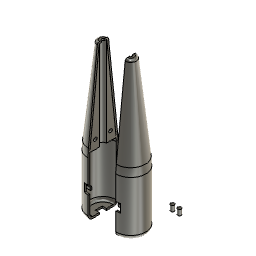
magic_wand_enclosure (Autodesk Fusion 360 design; units mm, degrees)
Autodesk Fusion 360 part; units mm, degrees
sketch "Sketch1" plane through (0, 0, 0) normal (0, 0, 1) x (1, 0, 0)
  circle A0 centre (0, 0) radius 19
  dimension "d1" = 38
  constraint coincident A0.centre origin
  measures "d1" diameter of A0
extrude "Extrude1" add sketch "Sketch1" along normal blind 82 makes body 1
sketch "Sketch2" plane through (0, 0, 82) normal (0, 0, 1) x (-1, 0, 0)
  circle A0 centre (0, 0) radius 19
  circle A1 centre (0, 0) radius 5
  dimension "d4" = 10
  constraint coincident A0.centre A1.centre
  measures "d4" diameter of A1
extrude "Extrude2" add sketch "Sketch2" along normal blind 128.5 contours A1 bodies 1
sketch "Sketch3" plane through (0, 0, 0) normal (0, 0, 1) x (1, 0, 0)
  circle A0 centre (70, 0) radius 19
  dimension "d7" = 38
  measures "d7" diameter of A0
extrude "Extrude3" add sketch "Sketch3" along normal blind 128.5 separate body makes body 2
sketch "Sketch4" plane through (0, 0, 128.5) normal (0, 0, 1) x (-1, 0, 0)
draft "Draft1" angle 6 neutral plane through (0, 0, 0) pull (0, 0, 1) 1 faces at (51.0944, 1.8918, 42.8333) on bodies 2
move_body "Move1" bodies 2 to x (1, 0, 0) y (0, 1, 0) z (0, 0, 1) at (-70, 0, 82)
combine "Combine1" operation add target body 2 tool bodies 1
fillet "Fillet1" radius 4 1 edges at (-17.7142, -6.8707, 0) on bodies 2
fillet "Fillet2" radius 0.8 1 edges at (-5.1223, -1.9868, 210.5) on bodies 2
fillet "Fillet3" radius 110 1 edges at (-17.7142, -6.8707, 82) on bodies 2
shell "Shell1" thickness 2.5 outward yes removed faces 0 bodies 2
sketch "Sketch5" plane through (0, 0, 0) normal (0, 0, 1) x (1, 0, 0)
  circle A0 centre (100, 0) radius 19
  dimension "d20" = 38
  measures "d20" diameter of A0
extrude "Extrude4" add sketch "Sketch5" along normal blind 128.5 separate body makes body 3
sketch "Sketch6" plane through (0, 0, 0) normal (0, 0, 1) x (1, 0, 0)
  circle A0 centre (150, 0) radius 5
  dimension "d23" = 10
  measures "d23" diameter of A0
extrude "Extrude5" add sketch "Sketch6" along normal blind 128.5 separate body makes body 4
move_body "Move2" bodies 4 to x (1, 0, 0) y (0, 1, 0) z (0, 0, 1) at (-50, 0, 0)
combine "Combine2" operation cut target body 3 tool bodies 4
draft "Draft2" angle 6 neutral plane through (0, 0, 0) pull (0, 0, 1) 1 faces at (81.0944, 1.8918, 42.8333) on bodies 3
move_body "Move3" bodies 3 to x (1, 0, 0) y (0, 1, 0) z (0, 0, 1) at (-100, 0, 81.5)
split "Split1" by plane through (0, 0, 0) normal (1, 0, 0) bodies 2 makes body 5 at (7.5898, 18.3035, 98.1655)
move_body "Move4" bodies 5 to x (1, 0, 0) y (0, 1, 0) z (0, 0, 1) at (70, 0, 0)
split "Split2" by plane through (0, 0, 0) normal (1, 0, 0) bodies 3 makes body 6 at (16.6383, 7.1249, 90.0667)
move_body "Move5" bodies 6 to x (1, 0, 0) y (0, 1, 0) z (0, 0, 1) at (70, 0, 0)
move_body "Move6" bodies 5 6 to x (1, 0, 0) y (0, 1, 0) z (0, 0, 1) at (-70, 0, 0)
sketch "Sketch7" plane through (0, 0, 213) normal (0, 0, 1) x (-1, 0, 0)
  line L0 (0, 4.7738) -> (0, -4.7738)
  arc A0 (0, -4.7738) -> (0, 4.7738) centre (0, 0) ccw
  circle A1 centre (0, 0) radius 2
  dimension "d28" = 4
  constraint coincident A0.centre A1.centre
  measures "d28" diameter of A1
extrude "Extrude6" cut sketch "Sketch7" against normal blind 4 contours L0 A1 picked at (-0.4534, -0.4887) bodies 5
sketch "Sketch8" plane through (0, 0, 213) normal (0, 0, 1) x (-1, 0, 0)
  line L0 (0, 4.7738) -> (0, -4.7738)
  arc A0 (0, -4.7738) -> (0, 4.7738) centre (0, 0) ccw
  circle A1 centre (0, 0) radius 2
  dimension "d31" = 4
  constraint concentric A0 A1
  measures "d31" diameter of A1
extrude "Extrude7" cut sketch "Sketch8" against normal blind 4 contours L0 A1 picked at (0.7193, 0.4836) bodies 2
sketch "Sketch9" plane through (0, 0, -2.5) normal (0, 0, -1) x (1, 0, 0)
  line L0 (0, -15) -> (0, 15)
  arc A0 (0, 15) -> (0, -15) centre (0, 0) ccw
  line L1 (6, 5) -> (-6, 5)
  line L2 (-6, 5) -> (-6, -5)
  line L3 (-6, -5) -> (6, -5)
  line L4 (6, -5) -> (6, 5)
  line L5 (6, 5) -> (-6, -5) construction
  line L6 (-6, 5) -> (6, -5) construction
  constraint horizontal L1
  constraint perpendicular L1 L2
  constraint parallel L1 L3
  constraint parallel L2 L4
  constraint coincident L5 A0.centre
  constraint coincident L6 A0.centre
  constraint coincident A0.centre origin
extrude "Extrude8" cut sketch "Sketch9" against normal blind 4 contours L0 L1 L2 L3 | L0 L1 L3 L4 bodies 2 5
sketch "Sketch10" plane through (0, 0, 0) normal (0, 0, 1) x (1, 0, 0)
  line L0 (45, 0) -> (57, 0)
  line L1 (57, 0) -> (57, 12)
  line L2 (57, 12) -> (45, 12)
  line L3 (45, 12) -> (45, 0)
  dimension "d36" = 12
  dimension "d37" = 12
  constraint horizontal L0
  constraint vertical L1
  constraint horizontal L2
  constraint vertical L3
  measures "d36" distance of L0.start L0.end
  measures "d37" distance of L0.start L2.end
extrude "Extrude9" add sketch "Sketch10" along normal blind 12 separate body makes body 7
move_body "Move7" bodies 7 to x (1, 0, 0) y (0, 1, 0) z (0, 0, 1) at (-51, 0, 20)
move_body "Move8" bodies 7 to x (1, 0, 0) y (0, 1, 0) z (0, 0, 1) at (0, -27, 10)
copy_body "CopyPasteBodies1" bodies 7 makes body 8
combine "Combine3" operation cut target body 5 tool bodies 7
combine "Combine4" operation cut target body 2 tool bodies 8
sketch "Sketch11" plane through (0, 0, 0) normal (0, 0, 1) x (1, 0, 0)
  line L0 (48, 8) -> (32, 8)
  line L1 (32, 8) -> (32, -8)
  line L2 (32, -8) -> (48, -8)
  line L3 (48, -8) -> (48, 8)
  line L4 (48, 8) -> (32, -8) construction
  line L5 (32, 8) -> (48, -8) construction
  point P0 (40, 0)
  dimension "d40" = 16
  dimension "d41" = 16
  constraint horizontal L0
  constraint perpendicular L0 L1
  constraint parallel L0 L2
  constraint parallel L1 L3
  constraint coincident L4 P0
  constraint coincident L5 P0
  measures "d40" distance of L1.end L2.end
  measures "d41" distance of L0.end L1.end
extrude "Extrude10" add sketch "Sketch11" along normal blind 2 separate body makes body 9
move_body "Move9" bodies 9 to x (1, 0, 0) y (0, 0, 1) z (0, -1, 0) at (0, -8, 8)
extrude "Extrude11" cut 1 faces at (42.6667, -9.3333, 16) along direction (0, 0, -1) blind 12 on bodies 9 bodies 9
move_body "Move10" bodies 9 to x (1, 0, 0) y (0, 1, 0) z (0, 0, 1) at (-40, -8.2, 34)
split "Split3" by plane through (0, 0, 0) normal (1, 0, 0) bodies 9 makes body 10 at (2.6667, -16.2, 36.6667)
move_body "Move11" bodies 5 6 10 to x (1, 0, 0) y (0, 1, 0) z (0, 0, 1) at (40, 0, 0)
sketch "Sketch13" plane through (0, 0, 0) normal (1, 0, 0) x (0, 1, 0)
  line L0 (-5.4941, 210) -> (-19, 81.5)
  line L1 (-19, 81.5) -> (-5, 81.5)
  line L2 (-5, 81.5) -> (-5, 210)
  line L3 (-5, 210) -> (-5.4941, 210)
  circle A0 centre (-11.0132, 94.0919) radius 2.5
  circle A1 centre (10.8183, 93.9651) radius 2.5
  dimension "d46" = 5
  dimension "d47" = 5
  measures "d46" diameter of A0
  measures "d47" diameter of A1
extrude "Extrude12" cut sketch "Sketch13" against normal blind 8 contours A0 | A1 bodies 3
combine "Combine5" operation add target body 9 tool bodies 3 2
combine "Combine6" operation add target body 5 tool bodies 6 10
sketch "Sketch14" plane through (0, 0, 0) normal (0, 0, 1) x (1, 0, 0)
  circle A0 centre (50, 50) radius 2.5
  dimension "d50" = 5
  measures "d50" diameter of A0
extrude "Extrude13" add sketch "Sketch14" along normal blind 8 separate body makes body 11
copy_body "CopyPasteBodies2" bodies 11 makes body 12
move_body "Move12" bodies 12 to x (1, 0, 0) y (0, 1, 0) z (0, 0, 1) at (10, 0, 0)
